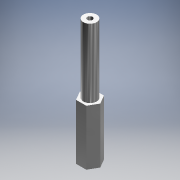
# Autodesk Inventor part: Roller drive shaft
Saved by Autodesk Inventor 2017 SP1 (Build 210196100, 196)
## iProperties
Created: 2018-02-02
Part Number: Roller drive shaft
Material: Aluminum 6061
Document SubType Name: Modeling
Designer: Ben
Density: 2.7 g/cm^3
Appearance: Chrome - Polished
Mass: 22.872 g
Surface Area: 41.0605 cm^2
Volume: 8.47111 cm^3
Author: Ben
Autodesk Inventor part; units mm, degrees
ref_plane "YZ Plane" through (0, 0, 0) normal (1, 0, 0) x (0, 1, 0)
ref_plane "XZ Plane" through (0, 0, 0) normal (0, 1, 0) x (-1, 0, 0)
ref_plane "XY Plane" through (0, 0, 0) normal (0, 0, 1) x (1, 0, 0)
sketch "Sketch1" plane through (0, 0, 0) normal (0, 1, 0) x (-1, 0, 0)
  line L0 (3.6662, -6.35) -> (-3.6662, -6.35)
  line L1 (-3.6662, -6.35) -> (-7.3323, 0)
  line L2 (-7.3323, 0) -> (-3.6662, 6.35)
  line L3 (-3.6662, 6.35) -> (3.6662, 6.35)
  line L4 (3.6662, 6.35) -> (7.3323, 0)
  line L5 (7.3323, 0) -> (3.6662, -6.35)
  point P0 (0, 0)
  point P1 (0, 0)
  dimension "d0" = 12.7
  constraints: 12 end point, 1 coincident, 1 horizontal, 13 other
  measures "d0" distance between parallel lines of L3 L0
extrude "Extrusion1" add sketch "Sketch1" against normal blind 39.6875
sketch "Sketch2" plane through (0, 0, 0) normal (0, 1, 0) x (1, 0, 0)
  circle A0 centre (0, 0) radius 4.7625
  dimension "d3" = 9.525
  constraints: 1 centre point, 1 coincident
  measures "d3" diameter of A0
extrude "Extrusion2" add sketch "Sketch2" along normal blind 49.2125
sketch "Sketch3" plane through (0, -39.6875, 0) normal (0, -1, 0) x (1, 0, 0)
  circle A0 centre (0, 0) radius 4.7625 projected
  circle A1 centre (0, 0) radius 1.905
  dimension "d7" = 3.81
  constraints: 1 centre point, 1 coincident
  measures "d7" diameter of A1
extrude "Extrusion3" cut sketch "Sketch3" against normal blind 25.4 contours A1
sketch "Sketch4" plane through (0, 49.2125, 0) normal (0, 1, 0) x (1, 0, 0)
  circle A0 centre (0, 0) radius 1.905 projected
extrude "Extrusion4" cut sketch "Sketch4" against normal blind 25.4
body "Solid1"
